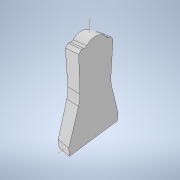
# Autodesk Inventor part: bearing holder
Saved by Autodesk Inventor 2021.1 (Build 251245000, 245)
## iProperties
Created: 2020-08-29
Part Number: bearing holder
Material: Generic
Document SubType Name: Sheet Metal
Designer: Vamshi
Density: 1 g/cm^3
Sheet Metal Rule: Default
Appearance: Default
Author: Vamshi
Autodesk Inventor part; units mm, degrees
ref_plane "YZ Plane" through (0, 0, 0) normal (1, 0, 0) x (0, 1, 0)
ref_plane "XZ Plane" through (0, 0, 0) normal (0, 1, 0) x (-1, 0, 0)
ref_plane "XY Plane" through (0, 0, 0) normal (0, 0, 1) x (1, 0, 0)
sketch "Sketch1" plane through (0, 0, 0) normal (0, 0, 1) x (1, 0, 0)
  line L0 (-116.84, -13.0015) -> (116.84, -13.0015)
  line L1 (116.84, -13.0015) -> (116.84, 25.0985)
  line L2 (-116.84, -13.0015) -> (-116.84, 25.0985)
  line L3 (0, -86.6615) -> (0, 428.9585) projected
  line L4 (-116.84, 25.0985) -> (-71.4229, 162.4275)
  line L5 (116.84, 25.0985) -> (71.4229, 162.4275)
  line L6 (-64.9999, 202.3045) -> (-64.9999, 324.8185)
  line L7 (64.9999, 202.3045) -> (64.9999, 324.8185)
  arc A0 (-65.1605, 181.3632) -> (-64.9999, 182.3601) centre (-68.1749, 182.3601) ccw
  arc A1 (-71.4229, 162.4275) -> (-64.9999, 202.3045) centre (-191.9999, 202.3045) ccw
  arc A2 (64.9999, 202.3045) -> (71.4229, 162.4275) centre (191.9999, 202.3045) ccw
  arc A3 (37.2472, 339.0425) -> (-37.2472, 339.0425) centre (0, 304.4985) ccw
  line L8 (-54.8399, 334.9785) -> (-46.559, 334.9785)
  line L9 (46.559, 334.9785) -> (54.8399, 334.9785)
  line L10 (0, 253.6985) -> (0, 227.7253)
  arc A4 (37.2472, 339.0425) -> (46.559, 334.9785) centre (46.559, 347.6785) ccw
  arc A5 (-46.559, 334.9785) -> (-37.2472, 339.0425) centre (-46.559, 347.6785) ccw
  arc A6 (37.2472, 339.0425) -> (46.559, 334.9785) centre (46.559, 347.6785) ccw
  line L11 (-54.8399, 334.9785) -> (-64.9999, 324.8185)
  line L12 (54.8399, 334.9785) -> (64.9999, 324.8185)
  point P0 (0, 0)
  point P1 (0, -13.0015)
  point P2 (-64.9999, 181.8487)
  point P3 (64.9999, 181.8487)
  point P4 (-64.9999, 334.9785)
  point P5 (64.9999, 334.9785)
  point P6 (-40.64, 334.9785)
  point P7 (40.64, 334.9785)
  dimension "d0" = 233.68
  dimension "d1" = 38.1
  dimension "d2" = 38.1
  dimension "d3" = 165.1
  dimension "d4" = 165.1
  dimension "d5" = 347.98
  dimension "d6" = 3.175
  dimension "d7" = 127
  dimension "d8" = 101.6
  dimension "d9" = 317.5
  dimension "d10" = 12.7
  dimension "d11" = 12.7
  dimension "d12" = 10.16
  dimension "d13" = 45
  dimension "d14" = 10.16
  dimension "d15" = 45
  constraints: 24 end point, 18 point on circle, 16 point on line, 12 tangent, 7 centre point, 3 horizontal, 3 vertical, 2 equal radius, 1 midpoint, 1 parallel, 1 perpendicular, 1 other
  measures "d0" distance of L0.start L0.end
  measures "d1" distance of L0.end L1.end
  measures "d2" distance of L0.start L2.end
  measures "d3" distance of L2.end point (-65, 181.849)
  measures "d4" distance of L1.end point (65, 181.849)
  measures "d5" distance from line of L0 point (-65, 334.979)
  measures "d6" radius of A0
  measures "d7" radius of A1
  measures "d8" diameter of A3
  measures "d9" distance from line of L0 A3.centre
  measures "d10" radius of A4
  measures "d11" radius of A5
  measures "d12" distance of L8.start point (-65, 334.979)
  measures "d13" angle of L8 L11
  measures "d14" distance of L9.end point (65, 334.979)
  measures "d15" angle of L9 L12
extrude "Extrusion1" add sketch "Sketch1" along normal mid plane 50.8
equation "\"d14\" = d12"
equation "\"d15\" = d13"
equation "\"BendRadius\" = Thickness"
equation "\"BendReliefWidth\" = Thickness"
equation "\"BendReliefDepth\" = 0.5 * Thickness"
equation "\"CornerReliefSize\" = 4 * Thickness"
equation "\"MinimumRemnant\" = 2 * Thickness"
equation "\"TransitionRadius\" = BendRadius"
equation "\"JacobiRadiusSize\" = BendRadius"
equation "\"GapSize\" = Thickness"
equation "\"Thickness\" = 3.048"
body "Solid1"
